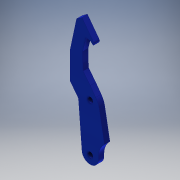
# Autodesk Inventor part: grip1a
Saved by Autodesk Inventor 2016 (Build 200138000, 138)
## iProperties
Created: 2016-01-10
Part Number: grip1a
Material: ABS Plastic
Document SubType Name: Modeling
Designer: Nanjar
Density: 1.06 g/cm^3
Appearance: Cool White(4)
Author: Nanjar
Autodesk Inventor part; units mm, degrees
ref_plane "YZ Plane" through (0, 0, 0) normal (1, 0, 0) x (0, 1, 0)
ref_plane "XZ Plane" through (0, 0, 0) normal (0, 1, 0) x (-1, 0, 0)
ref_plane "XY Plane" through (0, 0, 0) normal (0, 0, 1) x (1, 0, 0)
sketch "Sketch1" plane through (0, 0, 0) normal (0, 0, 1) x (1, 0, 0)
  circle A0 centre (0, 0) radius 1.5
  circle A1 centre (0, 26) radius 1.5
  arc A2 (-4.5, 0) -> (4.5, 0) centre (0, 0) ccw
  line L0 (4.5, 0) -> (4.5, 7.98)
  line L1 (-4.5, 0) -> (-6.4045, 23.6711)
  line L2 (-4.5, 0) -> (21.43, 0) construction
  line L3 (4.5, 7.98) -> (7.7584, 8.7295)
  line L4 (-1.4921, 25.8465) -> (17.6104, 25.8465) construction
  line L5 (-1.372, 54.3276) -> (-2.3083, 54.3276)
  line L6 (-4.5641, 62.9172) -> (-7.4382, 60.7619)
  line L7 (7.7584, 8.7295) -> (4.4705, 26.7439)
  line L8 (-0.0191, 32.9172) -> (4.4705, 26.7439)
  line L9 (0.2933, 53.9165) -> (-1.372, 54.3276)
  line L10 (-4.1293, 46.9816) -> (-4.1293, 41.4235)
  line L11 (-4.1293, 41.4235) -> (-3.8585, 37.8118)
  line L12 (-10.9822, 44.2097) -> (-10.9822, 29.6062)
  line L13 (2.3383, 53.7129) -> (1.6877, 52.735)
  line L14 (-7.4382, 60.7619) -> (-10.9822, 44.2097)
  line L15 (-2.3083, 54.3276) -> (-4.1293, 46.9816)
  line L16 (-6.4045, 23.6711) -> (-10.9822, 29.6062)
  line L17 (-0.0191, 32.9172) -> (-3.8585, 37.8118)
  line L18 (0.3525, 53.9019) -> (1.6877, 52.735)
  line L19 (2.3383, 53.7129) -> (-4.5641, 62.9172)
  line L20 (0.3525, 53.9019) -> (0.2933, 53.9165)
  dimension "d1" = 3
  dimension "d0" = 3
  dimension "d2" = 26
  dimension "d3" = 9
  dimension "d4" = 7.98
  dimension "d6" = 94.6
  constraints: 42 end point, 3 horizontal, 3 vertical, 2 centre point, 2 coincident, 2 point on circle, 2 point on line, 1 collinear, 1 perpendicular, 1 tangent, 3 other
  measures "d0" diameter of A0
  measures "d2" distance of point (0, 0) point (0, 26)
  measures "d3" diameter of A2
  measures "d4" distance of L0.start L0.end
  measures "d6" angle of L2 L1
extrude "Extrusion1" add sketch "Sketch1" along normal blind 3
fillet "Fillet1" radius 10 1 edges at (4.5, 7.98, 1.5)
fillet "Fillet6" radius 11 1 edges at (4.4705, 26.7439, 1.5)
fillet "Fillet7" radius 1.3 1 edges at (2.3383, 53.7129, 1.5)
body "Solid1"
